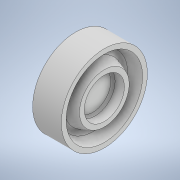
# Autodesk Inventor part: 711125
Saved by Autodesk Inventor 2022 (Build 260153000, 153)
## iProperties
Created: 2021-10-21
Part Number: 711125
Material: Типовые
Document SubType Name: Modeling
Designer: RaNSiD
Density: 1 g/cm^3
Appearance: По умолчанию
Mass: 37.8321 g
Surface Area: 122.044 cm^2
Volume: 37.8321 cm^3
Author: RaNSiD
Autodesk Inventor part; units mm, degrees
ref_plane "YZ Plane" through (0, 0, 0) normal (1, 0, 0) x (0, 1, 0)
ref_plane "XZ Plane" through (0, 0, 0) normal (0, 1, 0) x (-1, 0, 0)
ref_plane "XY Plane" through (0, 0, 0) normal (0, 0, 1) x (1, 0, 0)
sketch "Эскиз1" plane through (0, 0, 0) normal (0, 0, 1) x (1, 0, 0)
  line L0 (0, 0) -> (20, 0)
  line L1 (20, 0) -> (20, 30)
  line L2 (20, 30) -> (0, 30)
  line L3 (0, 30) -> (0, 0)
  dimension "d0" = 20
  dimension "d1" = 30
  constraints: 8 end point, 2 parallel, 1 horizontal, 1 perpendicular
  measures "d0" distance of L2.end L1.end
  measures "d1" distance of L1.end L0.end
revolve "Вращение1" add sketch "Эскиз1" angle 360 about axis through (0, 0, 0) along (1, 0, 0)
sketch "Эскиз2" plane through (0, 0, 0) normal (0, 0, 1) x (1, 0, 0)
  line L0 (0, 0) -> (3, 0)
  line L1 (3, 0) -> (3, 26)
  line L2 (3, 26) -> (0, 26)
  line L3 (0, 26) -> (0, 0)
  line L4 (12, 0) -> (20, 0)
  line L5 (20, 0) -> (20, 14)
  line L6 (20, 14) -> (13.5, 14)
  line L7 (12, 12.5) -> (12, 0)
  line L8 (0, -30) -> (0, 30) construction
  line L9 (20, -30) -> (20, 30) projected
  line L10 (20, 17.3239) -> (12.316, 20.1206)
  line L11 (20, 26.6761) -> (12.316, 23.8794)
  arc A0 (12.316, 23.8794) -> (12.316, 20.1206) centre (13, 22) ccw
  line L12 (20, 17.3239) -> (20, 26.6761)
  line L13 (0, 0) -> (20, 0)
  arc A1 (13.5, 14) -> (12, 12.5) centre (13.5, 12.5) ccw
  point P0 (12, 14)
  dimension "d3" = 3
  dimension "d4" = 26
  dimension "d5" = 8
  dimension "d6" = 14
  dimension "d7" = 20
  dimension "d8" = 2
  dimension "d9" = 70
  dimension "d11" = 22
  dimension "d12" = 7
  dimension "d14" = 1.5
  constraints: 24 end point, 5 point on line, 4 parallel, 4 point on circle, 4 tangent, 3 horizontal, 2 centre point, 2 perpendicular, 1 collinear, 1 equal length
  measures "d3" distance of L2.end L1.end
  measures "d4" distance of L1.end L0.end
  measures "d5" distance of point (12, 14) L5.end
  measures "d6" distance of L5.end L4.end
  measures "d7" distance from line of L8 L4.end
  measures "d8" radius of A0
  measures "d9" angle of L9 L10
  measures "d11" vertical distance of L0.start A0.centre
  measures "d12" horizontal distance of L10.start A0.centre
  measures "d14" radius of A1
revolve "Вращение2" cut sketch "Эскиз2" angle 360 about axis through (0, 0, 0) along (1, 0, 0)
